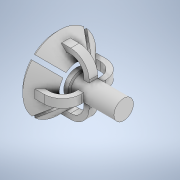
# Autodesk Inventor part: Weapon-Healing-Barrel
Saved by Autodesk Inventor 2020 (Build 240168000, 168)
## iProperties
Created: 2019-12-04
Part Number: Weapon-Healing-Barrel
Material: Generic
Document SubType Name: Modeling
Designer: Victor
Density: 1 g/cm^3
Appearance: Default
Author: Victor
Autodesk Inventor part; units mm, degrees
ref_plane "YZ Plane" through (0, 0, 0) normal (1, 0, 0) x (0, 1, 0)
ref_plane "XZ Plane" through (0, 0, 0) normal (0, 1, 0) x (-1, 0, 0)
ref_plane "XY Plane" through (0, 0, 0) normal (0, 0, 1) x (1, 0, 0)
sketch "Sketch1" plane through (0, 0, 0) normal (0, 0, 1) x (1, 0, 0)
  circle A0 centre (0, 0) radius 4.559
  dimension "d0" = 9.118
  constraints: 1 centre point, 1 coincident
  measures "d0" diameter of A0
extrude "Extrusion1" add sketch "Sketch1" along normal blind 20
sketch "Sketch3" plane through (0, 0, 20) normal (0, 0, 1) x (1, 0, 0)
  circle A0 centre (0, 0) radius 6
  dimension "d3" = 12
  constraints: 1 centre point, 1 coincident
  measures "d3" diameter of A0
extrude "Extrusion2" add sketch "Sketch3" along normal blind 2
sketch "Sketch4" plane through (0, 0, 0) normal (1, 0, 0) x (0, 1, 0)
  line L0 (7.1898, 22.9761) -> (15.6751, 31.4614)
  line L1 (7.1898, 22.9761) -> (19.1898, 22.9761) construction
  line L2 (15.6751, 31.4614) -> (17.0893, 30.0472)
  line L3 (17.0893, 30.0472) -> (8.604, 21.5619)
  line L4 (8.604, 21.5619) -> (7.1898, 22.9761)
  line L5 (6, 22) -> (-6, 22) projected
  line L6 (0, 36.5496) -> (0, 0)
  line L7 (-7.1898, 22.9761) -> (-15.6751, 31.4614)
  line L8 (-15.6751, 31.4614) -> (-17.0893, 30.0472)
  line L9 (-17.0893, 30.0472) -> (-8.604, 21.5619)
  line L10 (-8.604, 21.5619) -> (-7.1898, 22.9761)
  dimension "d6" = 12
  dimension "d7" = 45
  dimension "d8" = 2
  dimension "d9" = 0.9761
  dimension "d10" = 0.4381
  dimension "d11" = 2.604
  constraints: 20 end point, 4 symmetric about line, 2 perpendicular, 1 equal length, 1 horizontal, 1 vertical
  measures "d6" distance of L0.start L0.end
  measures "d7" angle of L1 L0
  measures "d8" distance of L0.end L2.end
  measures "d9" distance from line of L5 L0.start
  measures "d10" vertical distance of L5.start L3.end
  measures "d11" horizontal distance of L5.start L3.end
revolve "Revolution1" add sketch "Sketch4" angle 360 about axis through (0, 0, 36.5496) along (0, 0, -1) contours L0 L2 L3 L4
sketch "Sketch5" plane through (0, 0, 0) normal (0, 0, 1) x (1, 0, 0)
  circle A0 centre (0, 0) radius 17.0893
  circle A1 centre (0, 0) radius 17.0893 projected
  circle A2 centre (0, 0) radius 4.559 projected
  circle A3 centre (0, 0) radius 15.6751 projected
  line L0 (9.2517, 7.8375) -> (12.7911, 11.3768)
  line L1 (7.8375, 9.2517) -> (11.3768, 12.7911)
  line L2 (-7.8375, 9.2517) -> (-11.3768, 12.7911)
  line L3 (-9.2517, 7.8375) -> (-12.7911, 11.3768)
  line L4 (-9.2517, -7.8375) -> (-12.7911, -11.3768)
  line L5 (-7.8375, -9.2517) -> (-11.3768, -12.7911)
  line L6 (7.8375, -9.2517) -> (11.3768, -12.7911)
  line L7 (9.2517, -7.8375) -> (12.7911, -11.3768)
  line L8 (-4.3274, 5.7416) -> (-7.8375, 9.2517)
  line L9 (-5.7416, 4.3274) -> (-9.2517, 7.8375)
  line L10 (-5.7416, -4.3274) -> (-9.2517, -7.8375)
  line L11 (-4.3274, -5.7416) -> (-7.8375, -9.2517)
  line L12 (4.3274, -5.7416) -> (7.8375, -9.2517)
  line L13 (5.7416, -4.3274) -> (9.2517, -7.8375)
  line L14 (5.7416, 4.3274) -> (9.2517, 7.8375)
  line L15 (4.3274, 5.7416) -> (7.8375, 9.2517)
  arc A4 (5.7416, 4.3274) -> (4.3274, 5.7416) centre (0, 0) ccw
  arc A5 (-4.3274, 5.7416) -> (-5.7416, 4.3274) centre (0, 0) ccw
  arc A6 (-5.7416, -4.3274) -> (-4.3274, -5.7416) centre (0, 0) ccw
  arc A7 (4.3274, -5.7416) -> (5.7416, -4.3274) centre (0, 0) ccw
  point P0 (-12.7703, -11.3561)
  point P1 (-11.3561, -12.7703)
  point P2 (11.3561, -12.7703)
  point P3 (12.7703, -11.3561)
  point P4 (-12.7703, 11.3561)
  point P5 (-11.3561, 12.7703)
  point P6 (12.7703, 11.3561)
  point P7 (11.3561, 12.7703)
  constraints: 32 end point, 8 point on circle, 5 centre point, 2 coincident
extrude "Extrusion4" cut sketch "Sketch5" along normal blind 50 contours L0 A3 L1 A0 | A0 L6 A3 L7 | L0 L14 A4 L15 L1 A3 | A3 L6 L12 A7 L13 L7 | L2 A3 L3 A0 | A0 L4 A3 L5 | L2 L8 A5 L9 L3 A3 | A3 L4 L10 A6 L11 L5
sketch "Sketch6" plane through (0, 0, 0) normal (1, 0, 0) x (0, 1, 0)
  line L0 (11.2798, 27.0245) -> (14.4135, 27.0245)
  line L1 (14.4135, 27.0245) -> (14.4135, 24.5846)
  line L2 (14.4135, 24.5846) -> (11.2798, 24.5846)
  line L3 (11.2798, 24.5846) -> (11.2798, 27.0245)
  line L4 (17.0893, 30.0472) -> (8.604, 21.5619) projected
  line L5 (11.2798, 27.0245) -> (14.4135, 24.5846) construction
  line L6 (14.4135, 27.0245) -> (11.2798, 24.5846) construction
  line L7 (3.339, 14.15) -> (5.779, 14.15)
  line L8 (5.779, 14.15) -> (5.779, 16.59)
  line L9 (5.779, 16.59) -> (3.339, 16.59)
  line L10 (3.339, 16.59) -> (3.339, 14.15)
  line L11 (4.559, 0) -> (4.559, 20) projected
  line L12 (3.339, 14.15) -> (5.779, 16.59) construction
  line L13 (5.779, 14.15) -> (3.339, 16.59) construction
  arc A0 (5.779, 14.15) -> (14.4135, 22.7844) centre (5.779, 22.7844) ccw
  line L14 (14.4135, 22.7844) -> (14.4135, 24.5846)
  arc A1 (5.779, 16.59) -> (11.9735, 22.7844) centre (5.779, 22.7844) ccw
  line L15 (11.9735, 22.7844) -> (11.9735, 24.5846)
  point P0 (0, 0)
  point P1 (12.8466, 25.8046)
  point P2 (4.559, 15.37)
  point P3 (14.0666, 27.0245)
  point P4 (11.6267, 24.5846)
  point P5 (4.559, 16.59)
  point P6 (4.559, 14.15)
  dimension "d26" = 2.4399
  dimension "d27" = 2.44
  dimension "d28" = 2.44
  dimension "d29" = 2.44
  constraints: 28 end point, 5 midpoint, 4 parallel, 4 point on circle, 2 centre point, 2 horizontal, 2 perpendicular, 2 tangent, 1 point on line, 1 vertical, 1 other
  measures "d26" distance of L0.end L1.end
  measures "d27" distance of L9.end L8.end
  measures "d28" distance of L8.end L7.end
  measures "d29" radial gap between concentric circles of A0 A1
extrude "Extrusion5" add sketch "Sketch6" along normal mid plane 4 contours L0 L1 L2 L4 | L14 A0 L8 A1 L15 L2 | L7 L11 L9 L8
pattern_circular "Circular Pattern1" count 4 over 360 about axis through (0, 0, -10) along (0, 0, 1) of "Extrusion5"
body "Solid1"
